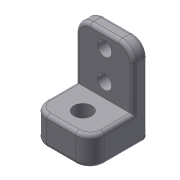
# Autodesk Inventor part: MainLiftBlock
Saved by Autodesk Inventor 2012 (Build 160160000, 160)
## iProperties
Created: 2013-01-16
Part Number: MainLiftBlock
Material: Aluminum-6061
Document SubType Name: Modeling
Designer: JesseK
Mass: 29.1534 g
Surface Area: 41.5099 cm^2
Volume: 10.7577 cm^3
Density: 2.71 g/cm^3
Author: JesseK
Autodesk Inventor part; units mm, degrees
ref_plane "YZ Plane" through (0, 0, 0) normal (1, 0, 0) x (0, 1, 0)
ref_plane "XZ Plane" through (0, 0, 0) normal (0, 1, 0) x (-1, 0, 0)
ref_plane "XY Plane" through (0, 0, 0) normal (0, 0, 1) x (1, 0, 0)
sketch "Sketch1" plane through (0, 0, 0) normal (0, 0, 1) x (1, 0, 0)
  line L0 (0, 0) -> (25.4, 0)
  line L1 (25.4, 0) -> (25.4, 38.1)
  line L2 (25.4, 38.1) -> (0, 38.1)
  line L3 (0, 38.1) -> (0, 0)
  dimension "d0" = 38.1
  dimension "d1" = 25.4
  constraints: 8 end point, 2 parallel, 1 horizontal, 1 perpendicular
  measures "d0" distance of L2.end L0.start
  measures "d1" distance of L0.start L0.end
extrude "Extrusion1" add sketch "Sketch1" along normal blind 25.4
sketch "Sketch4" plane through (25.4, 0, 0) normal (1, 0, 0) x (0, 0, -1)
  line L0 (0, 0) -> (-25.4, 0) projected
  line L1 (0, 0) -> (0, 38.1) projected
  line L2 (-25.4, 38.1) -> (-6.35, 38.1)
  line L3 (-6.35, 38.1) -> (-6.35, 12.7)
  line L4 (-6.35, 12.7) -> (-25.4, 12.7)
  line L5 (-25.4, 12.7) -> (-25.4, 38.1)
  dimension "d23" = 6.35
  dimension "d24" = 12.7
  constraints: 8 end point, 2 parallel, 1 horizontal, 1 perpendicular
  measures "d23" distance between parallel lines of L1 L3
  measures "d24" distance between parallel lines of L0 L4
extrude "Extrusion4" cut sketch "Sketch4" against normal through all
sketch "Sketch3" plane through (0, 0, 0) normal (0, 0, -1) x (-1, 0, 0)
  line L0 (-25.4, 38.1) -> (0, 38.1) projected
  line L1 (-25.4, 0) -> (-25.4, 38.1) projected
  circle A0 centre (-12.7, 31.75) radius 3.175
  circle A1 centre (-12.7, 19.05) radius 3.175
  dimension "d11" = 6.35
  dimension "d12" = 6.35
  dimension "d13" = 12.7
  dimension "d14" = 12.7
  dimension "d22" = 12.7
  constraints: 2 centre point, 1 equal radius
  measures "d11" diameter of A1
  measures "d12" distance from line of L0 A0.centre
  measures "d13" distance from line of L1 A1.centre
  measures "d14" distance from line of L1 A0.centre
  measures "d22" distance of A0.centre A1.centre
extrude "Extrusion3" cut sketch "Sketch3" against normal through all
sketch "Sketch5" plane through (0, 0, 0) normal (0, -1, 0) x (1, 0, 0)
  line L0 (25.4, 25.4) -> (0, 25.4) projected
  line L1 (25.4, 0) -> (25.4, 25.4) projected
  circle A0 centre (12.7, 15.875) radius 3.9688
  dimension "d27" = 9.525
  dimension "d28" = 7.9375
  dimension "d29" = 12.7
  constraints: 1 centre point
  measures "d27" distance from line of L0 A0.centre
  measures "d28" diameter of A0
  measures "d29" distance from line of L1 A0.centre
extrude "Extrusion5" cut sketch "Sketch5" against normal up to next
fillet "Fillet4" radius 1.5875 13 edges at (12.7, 38.1, 6.35) (12.7, 38.1, 0) (0, 25.4, 6.35) (0, 19.05, 0) (25.4, 25.4, 6.35) (25.4, 19.05, 0) (12.7, 0, 0) (25.4, 0, 12.7) (0, 0, 12.7) (25.4, 12.7, 15.875) (0, 12.7, 15.875) (12.7, 12.7, 25.4) (12.7, 0, 25.4)
fillet "Fillet5" radius 6.35 12 edges at (0.465, 12.235, 24.935) (0.465, 0.465, 24.935) (0, 6.35, 25.4) (24.935, 0.465, 24.935) (24.935, 12.235, 24.935) (25.4, 6.35, 25.4) (0.465, 37.635, 5.885) (0.465, 37.635, 0.465) (0, 38.1, 3.175) (24.935, 37.635, 5.885) (24.935, 37.635, 0.465) (25.4, 38.1, 3.175)
sketch "Sketch6" plane through (1.5875, 0, 1.5875) normal (0, -1, 0) x (1, 0, 0)
  circle A0 centre (2.7307, 5.3937) radius 0.4473
  point P0 (-1.5875, -1.5875)
  constraints: 1 centre point
extrude "Extrusion6" cut sketch "Sketch6" against normal blind 2.54
body "Solid1"
